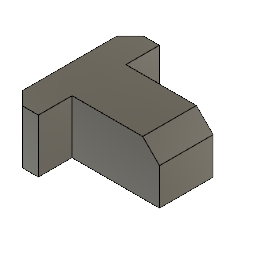
Jar tab (Autodesk Fusion 360 design; units mm, degrees)
Autodesk Fusion 360 part; units mm, degrees
sketch "Schizzo1" plane through (0, 0, 0) normal (0, 0, 1) x (1, 0, 0)
  line L0 (0, 0) -> (13, 0)
  line L1 (13, 0) -> (13, 8)
  line L2 (13, 8) -> (0, 8)
  line L3 (0, 8) -> (0, 0)
  line L4 (0, -5) -> (-4.3713, -5)
  line L5 (-4.3713, -5) -> (-4.3713, 13)
  line L6 (-4.3713, 13) -> (0, 13)
  line L7 (0, 13) -> (0, -5)
  dimension "d1" = 13
  dimension "d2" = 8
  dimension "d3" = 5
  dimension "d4" = 5
  constraint horizontal L0
  constraint vertical L1
  constraint horizontal L2
  constraint vertical L3
  constraint coincident L0.start L3.end
  constraint horizontal L4
  constraint vertical L5
  constraint horizontal L6
  constraint vertical L7
  measures "d1" distance of L0.start L0.end
  measures "d2" distance of L0.start L2.end
  measures "d3" distance of L2.end L6.end
  measures "d4" distance of L0.start L4.start
extrude "Estrusione1" add sketch "Schizzo1" along normal blind 6.5 makes body 1
chamfer "Smusso1" distance 3.5 angle 45 2 edges at (-4.3713, -5, 3.25) (-4.3713, 13, 3.25) on bodies 1
extrude "Estrusione2" add sketch "Schizzo1" along normal blind 8 separate body makes body 2
chamfer "Smusso2" distance 2 angle 45 2 edges at (-4.3713, -5, 4) (-4.3713, 13, 4) on bodies 2
chamfer "Smusso3" distance 2.5 angle 45 1 edges at (13, 4, 8) on bodies 2
hidden bodies 1
